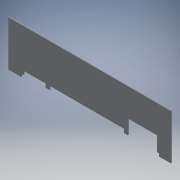
# Autodesk Inventor part: TSIWall
Saved by Autodesk Inventor 2017 (Build 210142000, 142)
## iProperties
Created: 2017-03-08
Part Number: TSIWall
Material: Generic
Document SubType Name: Modeling
Designer: hoeflinc
Density: 1 g/cm^3
Appearance: Default
Quantity: 1
Author: hoeflinc
Autodesk Inventor part; units mm, degrees
ref_plane "YZ Plane" through (0, 0, 0) normal (1, 0, 0) x (0, 1, 0)
ref_plane "XZ Plane" through (0, 0, 0) normal (0, 1, 0) x (-1, 0, 0)
ref_plane "XY Plane" through (0, 0, 0) normal (0, 0, 1) x (1, 0, 0)
sketch "Sketch1" plane through (0, 0, 0) normal (0, 0, 1) x (1, 0, 0)
  line L0 (0, 0) -> (454.025, 0)
  line L1 (454.025, 0) -> (454.025, 127)
  line L2 (454.025, 127) -> (0, 127)
  line L3 (0, 127) -> (0, 0)
  dimension "d0" = 127
  dimension "d1" = 454.025
  constraints: 8 end point, 2 parallel, 1 horizontal, 1 perpendicular
  measures "d0" distance of L2.end L0.start
  measures "d1" distance of L0.start L0.end
extrude "Extrusion1" add sketch "Sketch1" along normal blind 2.3622
sketch "Sketch2" plane through (0, 0, 2.3622) normal (0, 0, 1) x (1, 0, 0)
  line L0 (35.56, 0) -> (35.56, 8.128)
  line L1 (35.56, 8.128) -> (41.91, 8.128)
  line L2 (41.91, 8.128) -> (41.91, 18.288)
  line L3 (41.91, 18.288) -> (104.14, 18.288)
  line L4 (104.14, 18.288) -> (104.14, 8.128)
  line L5 (104.14, 8.128) -> (114.935, 8.128)
  line L6 (114.935, 8.128) -> (114.935, 18.288)
  line L7 (114.935, 18.288) -> (323.215, 18.288)
  line L8 (323.215, 18.288) -> (323.215, 8.128)
  line L9 (323.215, 8.128) -> (334.01, 8.128)
  line L10 (334.01, 8.128) -> (334.01, 48.768)
  line L11 (334.01, 48.768) -> (415.29, 48.768)
  line L12 (415.29, 48.768) -> (415.29, 8.128)
  line L13 (415.29, 8.128) -> (421.64, 8.128)
  line L14 (421.64, 8.128) -> (421.64, 0)
  line L15 (0, 127) -> (0, 0) projected
  line L16 (454.025, 0) -> (454.025, 127) projected
  line L17 (0, 0) -> (454.025, 0) projected
  line L18 (35.56, 0) -> (421.64, 0)
  dimension "d4" = 35.56
  dimension "d5" = 6.35
  dimension "d6" = 62.23
  dimension "d7" = 10.795
  dimension "d8" = 208.28
  dimension "d12" = 8.128
  dimension "d13" = 10.16
  dimension "d14" = 10.16
  dimension "d15" = 40.64
  dimension "d18" = 454.025
  dimension "d19" = 10.795
  dimension "d20" = 81.28
  dimension "d21" = 6.35
  constraints: 32 end point, 9 perpendicular, 6 point on line, 2 parallel, 1 collinear, 1 vertical
  measures "d4" distance between parallel lines of L15 L0
  measures "d5" distance of L0.end L1.end
  measures "d6" distance of L2.end L3.end
  measures "d7" distance of L4.end L5.end
  measures "d8" distance of L6.end L7.end
  measures "d12" distance between parallel lines of L17 L1
  measures "d13" distance of L1.end L2.end
  measures "d14" distance of L5.end L6.end
  measures "d15" distance of L11.end L12.end
  measures "d18" distance between parallel lines of L16 L15
  measures "d19" distance of L8.end L9.end
  measures "d20" distance of L10.end L11.end
  measures "d21" distance between parallel lines of L12 L14
extrude "Extrusion2" cut sketch "Sketch2" against normal blind 2.3622
body "Solid1"
